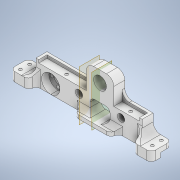
# Autodesk Inventor part: MotorBracketv2
Saved by Autodesk Inventor 2022 (Build 260153000, 153)
## iProperties
Created: 2022-01-31
Part Number: MotorBracketv2
Material: ABS プラスチック
Document SubType Name: Modeling
Designer: shiokaze
Density: 1.06 g/cm^3
Appearance: 滑らか - 白
Mass: 5.74152 g
Surface Area: 41.0545 cm^2
Volume: 5.41653 cm^3
Author: shiokaze
Autodesk Inventor part; units mm, degrees
ref_plane "YZ Plane" through (0, 0, 0) normal (1, 0, 0) x (0, 1, 0)
ref_plane "XZ Plane" through (0, 0, 0) normal (0, 1, 0) x (-1, 0, 0)
ref_plane "XY Plane" through (0, 0, 0) normal (0, 0, 1) x (1, 0, 0)
sketch "スケッチ2" plane through (0, 0, 0) normal (0, 0, 1) x (1, 0, 0)
  line L0 (-46.5, 12.5) -> (31.5, 12.5)
  line L1 (31.5, 12.5) -> (31.5, -12.5)
  line L2 (31.5, -12.5) -> (-46.5, -12.5)
  line L3 (-46.5, -12.5) -> (-46.5, 12.5)
  line L4 (-46.5, 12.5) -> (31.5, -12.5)
  line L5 (31.5, 12.5) -> (-46.5, -12.5)
  line L6 (-46.5, 12.5) -> (-9, 12.5)
  line L7 (-9, 12.5) -> (-9, -7.5)
  line L8 (-9, -7.5) -> (-46.5, -7.5)
  line L9 (-46.5, -7.5) -> (-46.5, 12.5)
  line L10 (31.5, 12.5) -> (6, 12.5)
  line L11 (6, 12.5) -> (6, -7.5)
  line L12 (6, -7.5) -> (31.5, -7.5)
  line L13 (31.5, -7.5) -> (31.5, 12.5)
  line L14 (-30.9, -7.5) -> (-36.5, -7.5)
  line L15 (-36.5, -7.5) -> (-36.5, 0.7)
  line L16 (-36.5, 0.7) -> (-9, 0.7)
  line L17 (-9, 0.7) -> (-9, -0.4808)
  line L18 (6, -7.5) -> (21.5, -7.5)
  line L19 (21.5, -7.5) -> (21.5, 0.7)
  line L20 (21.5, 0.7) -> (6, 0.7)
  line L21 (6, 0.7) -> (6, -7.5)
  line L22 (31.5, -12.5) -> (25.5, -12.5)
  line L23 (25.5, -12.5) -> (25.5, -10)
  line L24 (25.5, -10) -> (31.5, -10)
  line L25 (31.5, -10) -> (31.5, -12.5)
  line L26 (-7.5, 0) -> (0, 0)
  point P0 (-7.5, 0)
  point P1 (-9, 12.5)
  point P2 (-9, 0.7)
  point P3 (-46.5, -7.5)
  point P4 (31.5, -7.5)
  dimension "d0" = 78
  dimension "d1" = 25
  dimension "d15" = 37.5
  dimension "d16" = 5
  dimension "d17" = 25.5
  dimension "d18" = 6
  dimension "d19" = 2.5
  dimension "d20" = 10
  dimension "d21" = 10
  dimension "d22" = 11.8
  dimension "d26" = 7.5
  constraints: 54 end point, 12 parallel, 7 horizontal, 6 perpendicular, 4 collinear, 2 midpoint, 2 point on line, 1 coincident
  measures "d0" distance of L0.start L0.end
  measures "d1" distance of L0.end L1.end
  measures "d15" distance of L7.end L8.end
  measures "d16" distance between parallel lines of L2 L8
  measures "d17" distance of L12.end L11.end
  measures "d18" distance of L23.end L24.end
  measures "d19" distance of L22.end L23.end
  measures "d20" distance between parallel lines of L1 L19
  measures "d21" distance between parallel lines of L3 L15
  measures "d22" distance between parallel lines of L6 L16
  measures "d26" distance of L26.start L26.end
extrude "押し出し1" add sketch "スケッチ2" along normal blind 6 contours L0 L11 L5 L4 L7 | L8 L5 L3 | L16 L7 L4 | L4 L7 L5 L8 L15 L16 | L5 L8 L7 L4 L11 L12 L23 L2 | L4 L5 L7 | L11 L4 L5 | L5 L7 L8 | L1 L24 L23 L4 L12 | L20 L19 L12 L4 L11 | L4 L12 L11
sketch "スケッチ7" plane through (-9, 12.5, 0) normal (0, 1, 0) x (1, 0, 0)
  line L0 (0, 0) -> (-27.5, 0) projected
  line L1 (-27.5, 0) -> (-27.5, -6) projected
  line L2 (0, -6) -> (-27.5, -6) projected
  line L3 (0, 0) -> (0, -6) projected
  line L4 (30.5, 0) -> (15, 0) projected
  line L5 (15, 0) -> (15, -6) projected
  line L6 (30.5, -6) -> (15, -6) projected
  line L7 (30.5, 0) -> (30.5, -6) projected
  line L8 (0, -6) -> (-26, -6)
  line L9 (-26, -6) -> (-26, -1.5)
  line L10 (-26, -1.5) -> (0, -1.5)
  line L11 (0, -1.5) -> (0, -6)
  line L12 (15, -6) -> (29, -6)
  line L13 (29, -6) -> (29, -1.5)
  line L14 (29, -1.5) -> (15, -1.5)
  line L15 (15, -1.5) -> (15, -6)
  point P0 (9, 0)
  point P1 (29, -6)
  point P2 (-26, -6)
  dimension "d23" = 1.5
  dimension "d24" = 1.5
  dimension "d25" = 1.5
  constraints: 16 end point, 5 collinear, 4 parallel, 2 horizontal, 2 perpendicular
  measures "d23" distance between parallel lines of L7 L13
  measures "d24" distance between parallel lines of L4 L14
  measures "d25" distance between parallel lines of L1 L9
extrude "押し出し2" cut sketch "スケッチ7" against normal blind 1.6 from surface at -11.8 contours L3 L2 L9 L10 | L14 L13 L6 L5
sketch "スケッチ8" plane through (0, 0, 6) normal (0, 0, 1) x (1, 0, 0)
  circle A0 centre (-1.5, 6.35) radius 6.15 construction
  circle A1 centre (10, -4.4116) radius 9.6 construction
  circle A2 centre (-13, -4.4116) radius 9.6 construction
  circle A3 centre (-28.6303, -6.35) radius 6.15 construction
  line L0 (6, 12.5) -> (-9, 12.5) construction
  line L1 (6, 12.5) -> (-9, 12.5) construction
  line L2 (-46.5, -12.5) -> (25.5, -12.5) construction
  circle A4 centre (-13, -4.4116) radius 11
  circle A5 centre (10, -4.4116) radius 11
  line L3 (-2, -4.4116) -> (-1, -4.4116)
  line L4 (-13, -4.4116) -> (-1.5, 6.35) construction
  line L5 (-43.2356, 12.9995) -> (-27.4856, 12.9995) construction
  line L6 (-1.5, 6.35) -> (10, -4.4116) construction
  line L7 (-28.6303, -6.35) -> (-13, -4.4116) construction
  point P0 (0, 0)
  point P1 (-1.5, 12.5)
  point P2 (-1.5, 12.5)
  dimension "d29" = 12.3
  dimension "d123" = 22
  dimension "d124" = 22
  dimension "d30" = 19.2
  dimension "d31" = 19.2
  dimension "d32" = 12.3
  dimension "d132" = 1
  dimension "d144" = 15.75
  constraints: 10 end point, 5 coincident, 3 centre point, 3 equal length, 3 horizontal, 2 horizontal alignment, 2 midpoint, 2 point on line, 1 tangent, 1 vertical alignment, 6 other
  measures "d30" diameter of A2
  measures "d31" diameter of A1
  measures "d32" diameter of A3
  measures "d132" distance of L3.start L3.end
  measures "d144" distance of L5.start L5.end
hole "穴1" at (-13, -4.4116, 6) at (10, -4.4116, 6) direction (0, 0, -1) diameter 4 end through all
sketch "スケッチ9" plane through (0, 0, 6) normal (0, 0, 1) x (1, 0, 0)
  circle A0 centre (-1.5, 6.35) radius 6.15 construction
  circle A1 centre (10, -4.4116) radius 9.6 construction
  circle A2 centre (-13, -4.4116) radius 9.6 construction
  circle A3 centre (-28.4442, -7.5) radius 6.15 construction
  line L0 (6, 12.5) -> (-9, 12.5) projected
  line L1 (-46.5, -12.5) -> (25.5, -12.5) projected
  line L2 (6, 12.5) -> (-9, 12.5) projected
  circle A4 centre (-13, -4.4116) radius 11
  circle A5 centre (10, -4.4116) radius 11
  line L3 (-2, -4.4116) -> (-1, -4.4116)
  circle A6 centre (-28.4442, -7.5) radius 5
  line L4 (-46.5, -12.5) -> (25.5, -12.5) projected
  line L5 (-28.4442, -7.5) -> (-13, -4.4116)
  line L6 (-13, -4.4116) -> (-1.5, 6.35)
  line L7 (-1.5, 6.35) -> (10, -4.4116)
  line L8 (-17.7329, 13.873) -> (-33.4829, 13.873)
  point P0 (-1.5, 12.5)
  dimension "d42" = 12.3
  dimension "d127" = 22
  dimension "d128" = 22
  dimension "d43" = 19.2
  dimension "d44" = 19.2
  dimension "d45" = 12.3
  dimension "d131" = 1
  dimension "d133" = 10
  dimension "d145" = 15.75
  constraints: 10 end point, 6 coincident, 4 centre point, 3 equal length, 3 horizontal, 2 horizontal alignment, 2 point on line, 1 midpoint, 1 tangent, 1 vertical alignment, 6 other
  measures "d43" diameter of A2
  measures "d44" diameter of A1
  measures "d45" diameter of A3
  measures "d131" distance of L3.start L3.end
  measures "d133" diameter of A6
  measures "d145" distance of L8.start L8.end
hole "穴2" at (-1.5, 6.35, 6) direction (0, 0, -1) diameter 7 end through all
sketch "スケッチ10" plane through (0, 0, 6) normal (0, 0, 1) x (1, 0, 0)
  circle A0 centre (-13, -4.4116) radius 2 projected
  circle A1 centre (-13, -4.4116) radius 9.6 construction
  circle A2 centre (-28.4442, -7.5) radius 6.15 construction
  line L0 (-46.5, -12.5) -> (25.5, -12.5) projected
  line L1 (-46.5, -12.5) -> (25.5, -12.5) construction
  circle A3 centre (-28.4442, -7.5) radius 5
  line L2 (-28.4442, -7.5) -> (-13, -4.4116)
  line L3 (-38.1763, 8.069) -> (-22.4263, 8.069)
  dimension "d55" = 19.2
  dimension "d57" = 12.3
  dimension "d135" = 10
  dimension "d146" = 15.75
  constraints: 4 end point, 3 centre point, 3 coincident, 1 equal length, 1 horizontal, 1 tangent
  measures "d55" diameter of A1
  measures "d57" diameter of A2
  measures "d135" diameter of A3
  measures "d146" distance of L3.start L3.end
hole "穴3" at (-28.4442, -7.5, 6) direction (0, 0, -1) diameter 10 depth 4
sketch "スケッチ11" plane through (-28.4442, -7.5, 2) normal (0, 0, 1) x (1, 0, 0)
  circle A0 centre (0, 0) radius 5 projected
  point P0 (28.4442, 7.5)
  constraints: 1 coincident
hole "穴4" at (-28.4442, -7.5, 2) direction (0, 0, -1) diameter 4 depth 4
sketch "スケッチ12" plane through (-28.4442, -7.5, 2) normal (0, 0, 1) x (1, 0, 0)
  line L0 (0, 0) -> (0, 3.5)
  circle A0 centre (0, 0) radius 5 projected
  point P0 (28.4442, 7.5)
  point P1 (-3.5, 0)
  point P2 (0, -3.5)
  point P3 (3.5, 0)
  dimension "d72" = 3.5
  dimension "d75" = 360
  constraints: 2 coincident, 2 end point, 1 vertical, 5 other
  measures "d72" distance of L0.start L0.end
hole "穴5" at (-28.4442, -4, 2) at (-31.9442, -7.5, 2) at (-28.4442, -11, 2) at (-24.9442, -7.5, 2) direction (0, 0, -1) diameter 1.8 end through all clearance for "Countersunk Flat Head Screw ISO 2009/7046" size "M1.6" standard "ISO"
sketch "スケッチ14" plane through (0, 0, 6) normal (0, 0, 1) x (1, 0, 0)
  line L0 (-46.5, -7.5) -> (-46.5, -12.5) projected
  line L1 (-36.5, -7.5) -> (-46.5, -7.5) projected
  line L2 (-36.5, 0.7) -> (-36.5, -7.5) projected
  line L3 (-36.5, -7.5) -> (-46.5, -7.5) projected
  line L4 (-36.5, -7.5) -> (-36.5, -12.5)
  line L5 (-1.5, -10.5) -> (-1.5, -2.9)
  line L6 (-1.5, -2.9) -> (-7, -2.9)
  line L7 (-7, -2.9) -> (-7, -10.5)
  circle A0 centre (-1.5, 6.35) radius 3.5 projected
  line L8 (-1.5, -2.9) -> (4, -2.9)
  line L9 (4, -2.9) -> (4, -10.5)
  line L10 (-7, -10.5) -> (4, -10.5)
  line L11 (-46.5, -12.5) -> (25.5, -12.5) projected
  line L12 (-9, 12.5) -> (-9, -0.9) projected
  line L13 (-35, -0.9) -> (-9, -0.9) projected
  point P0 (0, 0)
  dimension "d84" = 2
  dimension "d85" = 2
  dimension "d86" = 2
  constraints: 14 end point, 2 symmetric about line, 1 horizontal, 1 midpoint, 1 parallel, 1 point on line, 1 vertical
  measures "d84" distance between parallel lines of L11 L10
  measures "d85" distance between parallel lines of L12 L7
  measures "d86" distance between parallel lines of L13 L6
extrude "押し出し3" cut sketch "スケッチ14" against normal through all contours L10 L7 L6 L5 | L5 L8 L9 L10
fillet "フィレット1" radius 4 4 edges at (-36.5, -7.5, 3) (21.5, -7.5, 3) (-9, 0.7, 0.75) (6, 0.7, 0.75)
fillet "フィレット2" radius 4 2 edges at (-9, 12.5, 3) (6, 12.5, 3)
fillet "フィレット3" radius 2.5 4 edges at (4, -10.5, 3) (4, -2.9, 3) (-7, -2.9, 3) (-7, -10.5, 3)
sketch "スケッチ16" plane through (0, 0, 6) normal (0, 0, 1) x (1, 0, 0)
  line L0 (4, -5.4) -> (4, -8) projected
  arc A0 (1.5, -10.5) -> (4, -8) centre (1.5, -8) ccw projected
  line L1 (1.5, -10.5) -> (-4.5, -10.5) projected
  arc A1 (-7, -8) -> (-4.5, -10.5) centre (-4.5, -8) ccw projected
  line L2 (-7, -8) -> (-7, -5.4) projected
  arc A2 (-4.5, -2.9) -> (-7, -5.4) centre (-4.5, -5.4) ccw projected
  line L3 (-4.5, -2.9) -> (1.5, -2.9) projected
  arc A3 (4, -5.4) -> (1.5, -2.9) centre (1.5, -5.4) ccw projected
  circle A4 centre (-28.4442, -7.5) radius 5 projected
  circle A5 centre (-1.5, 6.35) radius 3.5 projected
  circle A6 centre (-13, -4.4116) radius 2 projected
  circle A7 centre (10, -4.4116) radius 2 projected
  arc A8 (6, 8.5) -> (2, 12.5) centre (2, 8.5) ccw projected
  line L4 (2, 12.5) -> (-5, 12.5) projected
  arc A9 (-5, 12.5) -> (-9, 8.5) centre (-5, 8.5) ccw projected
  line L5 (-9, 8.5) -> (-9, -0.9) projected
  line L6 (-35, -0.9) -> (-9, -0.9) projected
  line L7 (-35, -0.9) -> (-35, 0.7) projected
  line L8 (-35, 0.7) -> (-36.5, 0.7) projected
  line L9 (-36.5, 0.7) -> (-36.5, -3.5) projected
  arc A10 (-40.5, -7.5) -> (-36.5, -3.5) centre (-40.5, -3.5) ccw projected
  line L10 (-40.5, -7.5) -> (-46.5, -7.5) projected
  line L11 (-46.5, -7.5) -> (-46.5, -12.5) projected
  line L12 (-46.5, -12.5) -> (-28.4442, -12.5) projected
  line L13 (25.5, -12.5) -> (25.5, -10) projected
  line L14 (25.5, -10) -> (31.5, -10) projected
  line L15 (31.5, -10) -> (31.5, -7.5) projected
  line L16 (31.5, -7.5) -> (25.5, -7.5) projected
  arc A11 (21.5, -3.5) -> (25.5, -7.5) centre (25.5, -3.5) ccw projected
  line L17 (21.5, -3.5) -> (21.5, 0.7) projected
  line L18 (21.5, 0.7) -> (20, 0.7) projected
  line L19 (20, 0.7) -> (20, -0.9) projected
  line L20 (6, -0.9) -> (20, -0.9) projected
  line L21 (6, -0.9) -> (6, 8.5) projected
  line L22 (-46.5, -7.5) -> (-46.5, -12.5) projected
  line L23 (-46.5, -12.5) -> (25.5, -12.5) projected
  line L24 (-46.5, -7.5) -> (-36.5, -7.5)
  line L25 (-36.5, -7.5) -> (-36.5, -12.5)
  line L26 (-36.5, -12.5) -> (-46.5, -12.5)
  line L27 (-46.5, -12.5) -> (-46.5, -7.5)
  line L28 (-28.4442, -12.5) -> (25.5, -12.5) projected
  point P0 (0, 0)
  constraints: 8 end point, 2 parallel, 1 collinear, 1 horizontal, 1 perpendicular, 1 point on line, 1 vertical alignment
extrude "押し出し4" add sketch "スケッチ16" along normal blind 10 from surface at -6 contours L12 L11 L10 L24 L25
sketch "スケッチ17" plane through (0, 0, 6) normal (0, 0, 1) x (1, 0, 0)
  line L0 (-36.5, -12.5) -> (25.5, -12.5) projected
  line L1 (8.5, -12.5) -> (-11.5, -12.5)
  line L2 (-11.5, -12.5) -> (-11.5, -10.5)
  line L3 (8.5, -10.5) -> (8.5, -12.5)
  line L4 (-11.5, -10.5) -> (8.5, -10.5)
  line L5 (1.5, -10.5) -> (-4.5, -10.5) projected
  line L6 (-4.5, -10.5) -> (1.5, -10.5) projected
  line L7 (-7, -8) -> (-7, -5.4) projected
  line L8 (4, -5.4) -> (4, -8) projected
  point P0 (0, 0)
  point P1 (-11.5, -12.5)
  point P2 (-1.5, -10.5)
  dimension "d119" = 20
  constraints: 8 end point, 3 parallel, 2 collinear, 2 midpoint, 1 point on line
  measures "d119" distance of L1.start L1.end
extrude "押し出し5" add sketch "スケッチ17" along normal blind 10 from surface at -6
fillet "フィレット4" radius 2.5 2 edges at (-11.5, -11.5, 6) (8.5, -11.5, 6)
fillet "フィレット5" radius 2.5 4 edges at (-8, -10.5, 6) (-12.75, -10.5, 6) (9.75, -10.5, 6) (5, -10.5, 6)
fillet "フィレット6" radius 2.5 2 edges at (-11.5, -11.5, 10) (8.5, -11.5, 10)
fillet "フィレット8" radius 2.5 2 edges at (-36.5, -10, 6) (-36.5, -10, 10)
fillet "フィレット9" radius 4 2 edges at (-35.25, -7.5, 6) (-38.5, -7.5, 6)
fillet "フィレット10" radius 2.5 2 edges at (-46.5, -10, 10) (-46.5, -10, 0)
sketch "スケッチ18" plane through (0, 0, 6) normal (0, 0, 1) x (1, 0, 0)
  line L0 (21.5, -3.5) -> (21.5, 0.7) projected
  line L1 (31.5, -10) -> (31.5, -7.5) projected
  line L2 (11, -12.5) -> (25.5, -12.5) projected
  line L3 (31.5, -12.5) -> (21.5, -12.5)
  line L4 (21.5, -12.5) -> (21.5, -7.5)
  line L5 (21.5, -7.5) -> (31.5, -7.5)
  line L6 (31.5, -7.5) -> (31.5, -12.5)
  line L7 (31.5, -7.5) -> (25.5, -7.5) projected
  point P0 (0, 0)
  constraints: 8 end point, 3 collinear, 2 parallel, 1 horizontal, 1 perpendicular, 1 point on line
extrude "押し出し6" add sketch "スケッチ18" along normal blind 5
fillet "フィレット11" radius 2.5 4 edges at (21.5, -10, 6) (21.5, -10, 11) (31.5, -10, 11) (31.5, -8.75, 0)
fillet "フィレット12" radius 5 2 edges at (20.2501, -7.5, 6) (23.5, -7.5, 6)
ref_plane "作業平面1" through (-7.5, -12.5, 6) normal (1, 0, 0) x (0, 0, -1)
ref_plane "作業平面2" through (-1.5, -8, 0) normal (-1, 0, 0) x (0, 0, 1)
sketch "スケッチ19" plane through (-40.5, -7.5, 10) normal (0, 1, 0) x (1, 0, 0)
  line L0 (-3, 2.5) -> (-3, 7.5)
  line L1 (-6, 7.5) -> (-6, 2.5) projected
  line L2 (-3.5, 0) -> (1.601, 0) projected
  line L3 (0, 10) -> (-3.5, 10) projected
  line L4 (-6, 7.5) -> (-6, 2.5) projected
  point P0 (40.5, 10)
  point P1 (0, 0)
  point P2 (-3, 5)
  point P3 (-6, 5)
  dimension "d107" = 3
  dimension "d108" = 5
  constraints: 2 coincident, 2 end point, 2 midpoint, 1 horizontal alignment, 1 vertical
  measures "d107" distance between parallel lines of L1 L0
  measures "d108" distance of L0.start L0.end
hole "穴6" at (-43.5, -7.5, 7.5) at (-43.5, -7.5, 2.5) direction (0, -1, 0) diameter 1.567 depth 0.1 tip angle 118 thread size "M2x0.4" class "6H" standard "ISO Metric profile"
mirror "ミラー1" about plane through (-7.5, -12.5, 6) normal (1, 0, 0) of "穴6"
sketch "スケッチ20" plane through (-9.101, -12.5, 10) normal (0, -1, 0) x (1, 0, 0)
  line L0 (0.101, -2.5) -> (15.101, -2.5)
  line L1 (15.101, -2.5) -> (15.101, -7.5)
  line L2 (15.101, -7.5) -> (0.101, -7.5)
  line L3 (0.101, -7.5) -> (0.101, -2.5)
  line L4 (0, 0) -> (15.202, 0) projected
  line L5 (7.601, -2.5) -> (7.601, 0)
  line L6 (11.101, -10) -> (4.101, -10) projected
  line L7 (7.601, -7.5) -> (7.601, -10)
  point P0 (9.101, -10)
  dimension "d116" = 15
  dimension "d117" = 5
  constraints: 12 end point, 4 midpoint, 2 parallel, 2 vertical, 1 collinear, 1 horizontal, 1 perpendicular, 1 vertical alignment
  measures "d116" distance of L1.end L2.end
  measures "d117" distance of L0.end L1.end
extrude "押し出し7" add sketch "スケッチ20" along normal blind 1.6
fillet "フィレット13" radius 2 4 edges at (-9, -13.3, 7.5) (6, -13.3, 7.5) (6, -13.3, 2.5) (-9, -13.3, 2.5)
sketch "スケッチ21" plane through (-5, 12.5, 0) normal (0, 1, 0) x (1, 0, 0)
  line L0 (25, -1.5) -> (25, -6) projected
  line L1 (11, -1.5) -> (25, -1.5) projected
  line L2 (11, -6) -> (11, -1.5) projected
  line L3 (11, -6) -> (25, -6) projected
  line L4 (-30, -6) -> (-30, -1.5) projected
  line L5 (-30, -6) -> (-4, -6) projected
  line L6 (-4, -1.5) -> (-4, -6) projected
  line L7 (-30, -1.5) -> (-4, -1.5) projected
  line L8 (25, -1.5) -> (25, -6) projected
  line L9 (25, -6) -> (11, -1.5)
  line L10 (-4, -6) -> (-30, -1.5)
  point P0 (5, 0)
  point P1 (-17, -3.75)
  point P2 (18, -3.75)
  constraints: 4 end point, 2 midpoint
hole "穴7" at (-22, 12.5, 3.75) at (13, 12.5, 3.75) direction (0, -1, 0) diameter 1.567 depth 13.5 tip angle 118 thread size "M2x0.4" class "6H" standard "ISO Metric profile"
